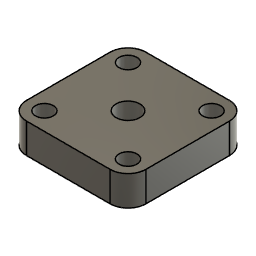
direct modeling - pe modified v2 (Autodesk Fusion 360 design; units mm, degrees)
Autodesk Fusion 360 part; units mm, degrees
sketch "Sketch1" plane through (0, 0, 0) normal (0, 1, 0) x (1, 0, 0)
  line L0 (50, -50) -> (-50, -50)
  line L1 (-50, -50) -> (-50, 50)
  line L2 (-50, 50) -> (50, 50)
  line L3 (50, 50) -> (50, -50)
  line L4 (50, -50) -> (-50, 50) construction
  line L5 (-50, -50) -> (50, 50) construction
  circle A0 centre (-35, 35) radius 7.5
  circle A1 centre (-35, -35) radius 7.5
  circle A2 centre (35, -35) radius 7.5
  circle A3 centre (35, 35) radius 7.5
  circle A4 centre (0, 0) radius 25
  dimension "d1" = 100
  dimension "d2" = 100
  dimension "d3" = 15
  dimension "d4" = 15
  dimension "d5" = 50
  constraint perpendicular L0 L1
  constraint parallel L0 L2
  constraint parallel L1 L3
  constraint horizontal L0
  constraint coincident L4 A4.centre
  constraint coincident L5 A4.centre
  constraint coincident A4.centre origin
  constraint coincident L4 A0.centre
  constraint coincident L5 A1.centre
  constraint coincident L4 A2.centre
  constraint coincident L5 A3.centre
  constraint horizontal A0.centre A3.centre
  constraint vertical A2.centre A3.centre
  constraint horizontal A1.centre A2.centre
  constraint equal A0 A3
  constraint equal A2 A3
  constraint equal A1 A2
  measures "d1" distance of L1.end L2.end
  measures "d2" distance of L0.end L1.end
  measures "d3" diameter of A0
  measures "d4" distance of L1 A0.centre
  measures "d5" diameter of A4
extrude "Extrude1" add sketch "Sketch1" along normal blind 25
fillet "Fillet1" radius 15 4 edges at (-50, 12.5, 50) (-50, 12.5, -50) (50, 12.5, 50) (50, 12.5, -50)
fillet "Fillet2" radius 12.5 1 edges at (-23.3082, 25, -9.0404)
chamfer "Chamfer1" distance 5 angle 45 8 edges at (-45.6066, 25, 45.6066) (0, 25, 50) (45.6066, 25, 45.6066) (50, 25, 0) (45.6066, 25, -45.6066) (0, 25, -50) (-45.6066, 25, -45.6066) (-50, 25, 0)
delete_face "DeleteFace1" 1 faces at (36.8593, 24.9858, 1.8396)
delete_face "DeleteFace2" 8 faces at (36.0894, 22.5, -47.4524) (-11.6667, 21.6667, -48.3333) (48.3333, 21.6667, -11.6667) (47.4524, 22.5, 36.0894) (11.6667, 21.6667, 48.3333) (-36.0894, 22.5, 47.4524) (-48.3333, 21.6667, 11.6667) (-47.4524, 22.5, -36.0894)
move_face "OffsetFaces1" offset 15 1 faces at (24.8758, 16.6667, -2.4892)
